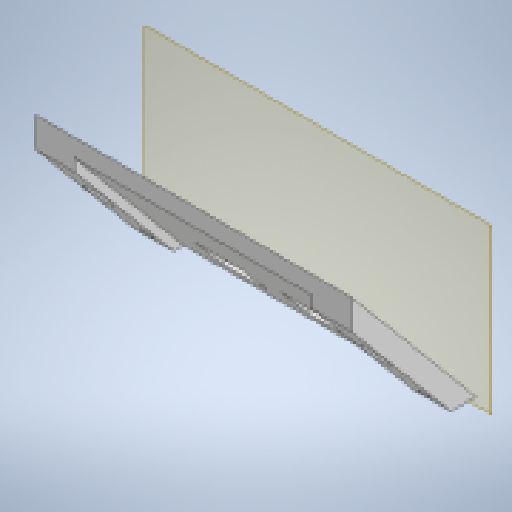
# Autodesk Inventor part: MS_Pokrywa
Saved by Autodesk Inventor 2023 (Build 270158000, 158)
## iProperties
Created: 2024-04-29
Part Number: MS_Pokrywa
Material: Ogólny
Document SubType Name: Modeling
Designer: kamil
Density: 1 g/cm^3
Appearance: Domyślna
Author: kamil
Autodesk Inventor part; units mm, degrees
ref_plane "YZ Plane" through (0, 0, 0) normal (1, 0, 0) x (0, 1, 0)
ref_plane "XZ Plane" through (0, 0, 0) normal (0, 1, 0) x (-1, 0, 0)
ref_plane "XY Plane" through (0, 0, 0) normal (0, 0, 1) x (1, 0, 0)
sketch "Szkic1" plane through (0, 0, 0) normal (1, 0, 0) x (0, 1, 0)
  line L0 (0, 0) -> (0, 3.916)
  line L1 (0, 3.916) -> (34.0032, 32.4481)
  line L2 (0, 0) -> (34.0032, 28.5321)
  line L3 (34.0032, 28.5321) -> (38.6701, 32.4481)
  line L4 (34.0032, 32.4481) -> (38.6701, 32.4481)
  dimension "d0" = 3.916
  dimension "d1" = 130
  dimension "d2" = 44.388
  constraints: 10 end point, 1 collinear, 1 horizontal, 1 horizontal alignment, 1 parallel, 1 vertical
  measures "d0" distance of L0.start L0.end
  measures "d1" angle of L0 L1
  measures "d2" distance of L0.end L1.end
extrude "Wyciągnięcie proste1" add sketch "Szkic1" against normal blind 82
sketch "Szkic2" plane through (0, 0, 0) normal (0, 0.6427876, -0.7660444) x (-1, 0, 0)
  circle A0 centre (5, 7.1954) radius 2.85 projected
  circle A1 centre (77, 7.1954) radius 2.85 projected
  point P0 (0, 0)
move faces "Przesuń1" translate (0, -1.2856, 1.5321) faces at (-27.3333, 22.6688, 22.9374)
sketch "Szkic3" plane through (-82, 30.8917, 32.4481) normal (0, -0.6427876, 0.7660444) x (1, 0, 0)
  line L0 (82, 5.9586) -> (82, 0) projected
  line L1 (82, 5.9586) -> (0, 5.9586) projected
  line L2 (0, 0) -> (0, 5.9586) projected
  line L3 (82, 0) -> (0, 0) projected
  line L4 (82, 0) -> (82, -40.3263) projected
  line L5 (82, 0) -> (0, 0) projected
  line L6 (0, -40.3263) -> (0, 0) projected
  line L7 (82, -40.3263) -> (0, -40.3263) projected
  line L8 (82, -40.3263) -> (82, -44.5216) projected
  line L9 (82, -40.3263) -> (0, -40.3263) projected
  line L10 (0, -44.5216) -> (0, -40.3263) projected
  line L11 (82, -44.5216) -> (0, -44.5216) projected
  line L12 (10, 5.9586) -> (72, 5.9586)
  line L13 (72, 5.9586) -> (72, -44.5216)
  line L14 (72, -44.5216) -> (10, -44.5216)
  line L15 (10, -44.5216) -> (10, 5.9586)
  point P0 (0, -20.1631)
  point P1 (10, -44.5216)
  point P2 (72, 5.9586)
  dimension "d9" = 10
  dimension "d10" = 10
  constraints: 8 end point, 2 parallel, 2 point on line, 1 horizontal, 1 midpoint, 1 perpendicular
  measures "d9" distance between parallel lines of L4 L13
  measures "d10" distance from line of L15 point (0, -20.163)
extrude "Wyciągnięcie proste2" cut sketch "Szkic3" against normal blind 2 contours L13 L3 L15 L1 | L13 L7 L15 L3 | L13 L11 L15 L7
hole "Otwór1" at (-5, 5.512, 4.6251) at (-77, 5.512, 4.6251) direction (0, -0.6427876, 0.7660444) diameter 3.2 depth 4.9998 counterbore diameter 5.7 counterbore depth 3.1
sketch "Szkic4" plane through (-82, 38.6701, 32.4481) normal (0, 0, 1) x (1, 0, 0)
  circle A0 centre (77, -21.1701) radius 3 projected
  circle A1 centre (5, -21.1701) radius 3 projected
  point P0 (82, -38.6701)
extrude "Wyciągnięcie proste3" cut sketch "Szkic4" against normal through all
ref_plane "Płaszczyzna konstrukcyjna1" through (0, 0, 0) normal (0, 0, 1) x (-1, 0, 0)
sketch "Szkic5" plane through (0, 0, 0) normal (0, 0, 1) x (-1, 0, 0)
  line L0 (30.5, -7.2) -> (26.1, -7.2) projected
  line L1 (26.1, -7.2) -> (26.1, -9.6) projected
  line L2 (26.1, -9.6) -> (30.5, -9.6) projected
  line L3 (30.5, -9.6) -> (30.5, -7.2) projected
  line L4 (51.5, -9.6) -> (51.5, -7.2) projected
  line L5 (55.9, -9.6) -> (51.5, -9.6) projected
  line L6 (51.5, -7.2) -> (55.9, -7.2) projected
  line L7 (55.9, -7.2) -> (55.9, -9.6) projected
  line L8 (35.8, -13.1) -> (25.1, -13.1) projected
  line L9 (46.2, -13.1) -> (56.9, -13.1) projected
  line L10 (24.1, -11.6) -> (24.1, -5.2)
  line L11 (24.1, -5.2) -> (32.5, -5.2)
  line L12 (32.5, -5.2) -> (32.5, -11.6)
  line L13 (32.5, -11.6) -> (24.1, -11.6)
  line L14 (24.1, -13.1) -> (35.8, -13.1)
  line L15 (35.8, -13.1) -> (35.8, -5.2)
  line L16 (35.8, -5.2) -> (24.1, -5.2)
  line L17 (24.1, -5.2) -> (24.1, -13.1)
  line L18 (49.5, -5.2) -> (49.5, -11.6)
  line L19 (49.5, -11.6) -> (57.9, -11.6)
  line L20 (57.9, -11.6) -> (57.9, -5.2)
  line L21 (57.9, -5.2) -> (49.5, -5.2)
  line L22 (57.9, -5.2) -> (46.2, -5.2)
  line L23 (46.2, -5.2) -> (46.2, -13.1)
  line L24 (46.2, -13.1) -> (57.9, -13.1)
  line L25 (57.9, -13.1) -> (57.9, -5.2)
  point P0 (0, 0)
  dimension "d23" = 2
  dimension "d24" = 2
  constraints: 32 end point, 4 parallel, 2 horizontal, 2 perpendicular, 1 point on line, 6 other
  measures "d23" distance between parallel lines of L1 L10
  measures "d24" distance between parallel lines of L4 L18
extrude "Wyciągnięcie proste4" cut sketch "Szkic5" along normal blind 15 contours L3 L2 L1 L0 | L4 L6 L7 L5 | L8 L14 L17 L13 L12 L16 L15 | L12 L13 L10 L11 | L23 L22 L18 L19 L25 L24 L9 | L21 L20 L19 L18
